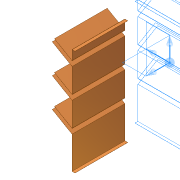
# Autodesk Inventor part: FeederMockup
Saved by Autodesk Inventor 2012 (Build 160160000, 160)
## iProperties
Created: 2013-01-12
Part Number: FeederMockup
Material: Default
Document SubType Name: Modeling
Designer: JesseK
Surface Area: 71892.1 cm^2
Volume: 5687.35 cm^3
Author: JesseK
Autodesk Inventor part; units mm, degrees
ref_plane "YZ Plane" through (0, 0, 0) normal (1, 0, 0) x (0, 1, 0)
ref_plane "XZ Plane" through (0, 0, 0) normal (0, 1, 0) x (-1, 0, 0)
ref_plane "XY Plane" through (0, 0, 0) normal (0, 0, 1) x (1, 0, 0)
sketch "Sketch2" plane through (0, 0, 0) normal (0, 0, 1) x (1, 0, 0)
  line L0 (0, 0) -> (0, 1828.8)
  line L1 (0, 1828.8) -> (-50.8, 1828.8)
  line L2 (-50.8, 1828.8) -> (-50.8, 1662.7882)
  line L3 (-50.8, 1662.7882) -> (-355.6, 1838.7645)
  line L4 (-355.6, 1838.7645) -> (-393.7, 1772.7734)
  line L5 (-393.7, 1772.7734) -> (-50.8, 1574.8)
  line L6 (-50.8, 1574.8) -> (-50.8, 1154.7882)
  line L7 (-50.8, 1154.7882) -> (-355.6, 1330.7645)
  line L8 (-355.6, 1330.7645) -> (-393.7, 1264.7734)
  line L9 (-393.7, 1264.7734) -> (-50.8, 1066.8)
  line L10 (-50.8, 1066.8) -> (-50.8, 646.7882)
  line L11 (-50.8, 646.7882) -> (-355.6, 822.7645)
  line L12 (-355.6, 822.7645) -> (-393.7, 756.7734)
  line L13 (-393.7, 756.7734) -> (-50.8, 558.8)
  line L14 (-50.8, 558.8) -> (-50.8, 0)
  line L15 (-50.8, 0) -> (0, 0)
  dimension "d0" = 60
  dimension "d1" = 558.8
  dimension "d3" = 304.8
  dimension "d4" = 1828.8
  dimension "d6" = 76.2
  dimension "d7" = 50.8
  dimension "d8" = 1574.8
  dimension "d10" = 1066.8
  constraints: 32 end point, 6 parallel, 6 perpendicular, 5 vertical, 3 collinear, 2 horizontal
  measures "d0" angle of L10 L11
  measures "d1" vertical distance of L0.start L13.end
  measures "d3" horizontal distance of L10.end L11.end
  measures "d4" distance of L0.start L0.end
  measures "d6" distance of L3.end L4.end
  measures "d7" distance of L14.end L0.start
  measures "d8" vertical distance of L0.start L5.end
  measures "d10" vertical distance of L0.start L9.end
extrude "Extrusion1" add sketch "Sketch2" along normal blind 914.4
shell "Shell1" thickness 1.5875 removed faces 6 at (-368.3, 800.7675, 304.8) at (-368.3, 1308.7675, 304.8) at (-368.3, 1816.7675, 304.8) at (0, 609.6, 304.8) at (-16.9333, 795.8667, 914.4) at (-16.9333, 795.8667, 0)
body "Solid1"
